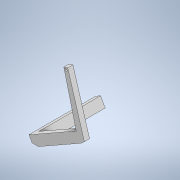
# Autodesk Inventor part: grip - C2-1
Saved by Autodesk Inventor 2021 (Build 250183000, 183)
## iProperties
Created: 2021-05-09
Part Number: grip - C2-1
Material: Generic
Document SubType Name: Modeling
Designer: Alsayaary
Density: 1 g/cm^3
Appearance: Default
Author: Abdulrahman
Autodesk Inventor part; units mm, degrees
ref_plane "YZ Plane" through (0, 0, 0) normal (1, 0, 0) x (0, 1, 0)
ref_plane "XZ Plane" through (0, 0, 0) normal (0, 1, 0) x (-1, 0, 0)
ref_plane "XY Plane" through (0, 0, 0) normal (0, 0, 1) x (1, 0, 0)
sketch "Sketch1" plane through (0, 0, 0) normal (0, 0, 1) x (1, 0, 0)
  circle A0 centre (152.0025, 356.0058) radius 5
  line L0 (28.751, 0) -> (220.0553, 108.6482)
  line L1 (220.0553, 108.6482) -> (233.0937, 120.8954)
  line L2 (233.0937, 120.8954) -> (159.1798, 368.1207)
  line L3 (159.1798, 368.1207) -> (141.7433, 362.9081)
  line L4 (141.7433, 362.9081) -> (196.9837, 143.9375)
  line L5 (196.9837, 143.9375) -> (-13.7687, 24.2435)
  line L6 (0, 0) -> (-13.7687, 24.2435)
  line L7 (0, 0) -> (28.751, 0)
  dimension "CHAMFER" = 28.751
  dimension "d1" = 60.406
  dimension "d2" = 29.594
  dimension "ARM_L" = 220.004
  dimension "ARM_L2" = 242.37
  dimension "ARM_VER_L" = 258.038
  dimension "ARM_VER_L2" = 225.831
  dimension "ARM_W2" = 18.199
  dimension "ARM_W" = 42.162
  dimension "PIN_HOLE" = 10
  dimension "d10" = 233.0937
  dimension "d11" = 120.8954
  dimension "d12" = 24.2435
  dimension "d13" = 13.7687
  dimension "d14" = 196.9837
  dimension "d15" = 220.0553
  dimension "d16" = 159.1798
  dimension "d17" = 152.0025
  dimension "d18" = 356.0058
  constraints: 16 end point, 1 centre point
  measures "CHAMFER" distance of L6.start L0.start
  measures "d1" angle of L7 L6
  measures "d2" angle of L7 L0
  measures "ARM_L" distance of L0.start L0.end
  measures "ARM_L2" distance of L4.end L5.end
  measures "ARM_VER_L" distance of L1.end L2.end
  measures "ARM_VER_L2" distance of L3.end L4.end
  measures "ARM_W2" distance of L2.end L3.end
  measures "ARM_W" distance of L0.end L4.end
  measures "PIN_HOLE" diameter of A0
  measures "d10" horizontal distance of point (0, 0) L1.end
  measures "d11" vertical distance of point (0, 0) L1.end
  measures "d12" vertical distance of point (0, 0) L5.end
  measures "d13" horizontal distance of point (0, 0) L5.end
  measures "d14" horizontal distance of point (0, 0) L4.end
  measures "d15" horizontal distance of point (0, 0) L0.end
  measures "d16" horizontal distance of point (0, 0) L2.end
  measures "d17" horizontal distance of L6.start A0.centre
  measures "d18" vertical distance of point (0, 0) A0.centre
extrude "Extrusion1" add sketch "Sketch1" along normal mid plane 23
sketch "Sketch2" plane through (0, 0, -11.5) normal (0, 0, -1) x (-1, 0, 0)
  line L0 (-7.9703, 36.5899) -> (13.7687, 24.2435)
  line L1 (13.7687, 24.2435) -> (-0.054, -0.0951)
  line L2 (0, 0) -> (-0.054, -0.0951)
  line L3 (0, 0) -> (-28.751, 0)
  line L4 (-7.9703, 36.5899) -> (-28.751, 0)
  line L5 (0, 0) -> (13.7687, 24.2435) projected
  line L6 (13.7687, 24.2435) -> (-196.9837, 143.9375) projected
  line L7 (-28.751, 0) -> (0, 0) projected
  point P0 (226.376, 276)
  constraints: 10 end point, 4 collinear, 1 parallel
extrude "Extrusion2" add sketch "Sketch2" along normal blind 274
sketch "Sketch3" plane through (196.9837, 143.9375, 11.5) normal (-0.4938, 0.8695, 0) x (0.8695, 0.4938, 0)
  line L0 (-242.3701, 0) -> (-217.3697, 0) projected
  line L1 (-242.3701, 0) -> (-241.6771, 0)
  line L2 (-241.6771, 0) -> (-241.6771, 63.016)
  line L3 (-241.6771, 63.016) -> (-242.3701, 63.016)
  line L4 (-242.3701, 63.016) -> (-242.3701, 0)
  point P0 (-242.3701, 11.5)
  point P1 (-241.6771, 0)
  dimension "d23" = 63.016
  dimension "d24" = 0.693
  constraints: 8 end point, 2 parallel, 1 horizontal, 1 perpendicular
  measures "d23" distance of L3.end L0.start
  measures "d24" distance of L2.end L3.end
extrude "Extrusion3" cut sketch "Sketch3" against normal blind 274
body "Solid1"
